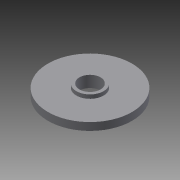
# Autodesk Inventor part: Y_tensioner_washer
Saved by Autodesk Inventor 2013 (Build 170138000, 138)
## iProperties
Created: 2014-02-03
Part Number: Y_tensioner_washer
Material: Ogólny
Document SubType Name: Modeling
Designer: Piotr
Density: 1 g/cm^3
Author: Piotr
Autodesk Inventor part; units mm, degrees
ref_plane "YZ Plane" through (0, 0, 0) normal (1, 0, 0) x (0, 1, 0)
ref_plane "XZ Plane" through (0, 0, 0) normal (0, 1, 0) x (-1, 0, 0)
ref_plane "XY Plane" through (0, 0, 0) normal (0, 0, 1) x (1, 0, 0)
sketch "Szkic1" plane through (0, 0, 0) normal (0, 0, 1) x (1, 0, 0)
  circle A0 centre (0, 0) radius 11
  circle A1 centre (0, 0) radius 2.75
  circle A2 centre (0, 0) radius 3.55
  dimension "d0" = 22
  dimension "d1" = 5.5
  dimension "d2" = 7.1
  constraints: 3 centre point, 3 coincident
  measures "d0" diameter of A0
  measures "d1" diameter of A1
  measures "d2" diameter of A2
extrude "Wyciągnięcie proste1" add sketch "Szkic1" along normal blind 3 contours A2
extrude "Wyciągnięcie proste2" add sketch "Szkic1" along normal blind 2 contours A0
